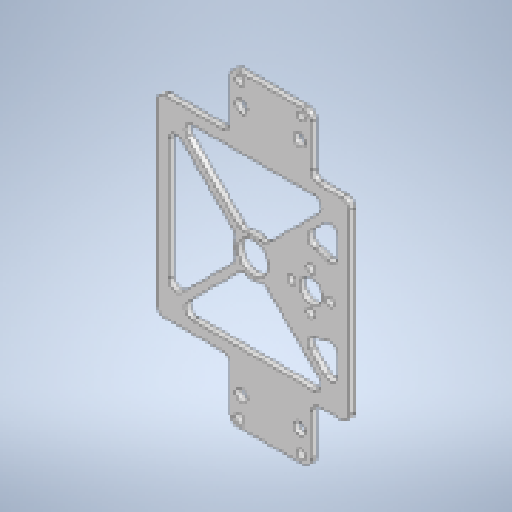
# Autodesk Inventor part: kataue
Saved by Autodesk Inventor 2025.1 (Build 291241000, 241)
## iProperties
Created: 2024-09-02
Part Number: kataue
Material: アルミニウム 2014-T4
Document SubType Name: Modeling
Designer: right
Density: 2.8 g/cm^3
Appearance: サテン
Mass: 6.17041 g
Surface Area: 41.087 cm^2
Volume: 2.20372 cm^3
Author: right
Autodesk Inventor part; units mm, degrees
ref_plane "YZ Plane" through (0, 0, 0) normal (1, 0, 0) x (0, 1, 0)
ref_plane "XZ Plane" through (0, 0, 0) normal (0, 1, 0) x (-1, 0, 0)
ref_plane "XY Plane" through (0, 0, 0) normal (0, 0, 1) x (1, 0, 0)
sketch "スケッチ1" plane through (0, 0, 0) normal (0, 0, 1) x (1, 0, 0)
  arc A0 (6.4508, -24.0185) -> (7.2151, -22.4459) centre (5.2151, -22.4459) ccw projected
  line L0 (7.2151, -22.4459) -> (7.2151, -18.7355) projected
  arc A1 (7.0743, -7.2531) -> (7.2151, -18.7355) centre (12.7151, -12.926) ccw projected
  arc A2 (7.0743, -7.2531) -> (2.2151, -6.426) centre (4.7151, -6.426) ccw projected
  line L1 (2.2151, -6.426) -> (2.2151, -154.426) projected
  arc A3 (2.2151, -154.426) -> (7.0743, -153.5989) centre (4.7151, -154.426) ccw projected
  arc A4 (7.2151, -142.1165) -> (7.0743, -153.5989) centre (12.7151, -147.926) ccw projected
  line L2 (7.2151, -142.1165) -> (7.2151, -138.4062) projected
  arc A5 (7.2151, -138.4062) -> (6.4508, -136.8336) centre (5.2151, -138.4062) ccw projected
  arc A6 (5.6865, -135.261) -> (6.4508, -136.8336) centre (7.6865, -135.261) ccw projected
  line L3 (5.6865, -135.261) -> (5.6865, -131.591) projected
  arc A7 (6.4508, -130.0185) -> (5.6865, -131.591) centre (7.6865, -131.591) ccw projected
  arc A8 (6.4508, -130.0185) -> (7.2151, -128.4459) centre (5.2151, -128.4459) ccw projected
  line L4 (7.2151, -128.4459) -> (7.2151, -122.426) projected
  arc A9 (9.2151, -120.426) -> (7.2151, -122.426) centre (9.2151, -122.426) ccw projected
  line L5 (9.2151, -120.426) -> (21.2151, -120.426) projected
  arc A10 (21.2151, -120.426) -> (23.2151, -118.426) centre (21.2151, -118.426) ccw projected
  line L6 (23.2151, -118.426) -> (23.2151, -42.426) projected
  arc A11 (23.2151, -42.426) -> (21.2151, -40.426) centre (21.2151, -42.426) ccw projected
  line L7 (21.2151, -40.426) -> (9.2151, -40.426) projected
  arc A12 (7.2151, -38.426) -> (9.2151, -40.426) centre (9.2151, -38.426) ccw projected
  line L8 (7.2151, -38.426) -> (7.2151, -32.4062) projected
  arc A13 (7.2151, -32.4062) -> (6.4508, -30.8336) centre (5.2151, -32.4062) ccw projected
  arc A14 (5.6865, -29.261) -> (6.4508, -30.8336) centre (7.6865, -29.261) ccw projected
  line L9 (5.6865, -29.261) -> (5.6865, -25.591) projected
  arc A15 (6.4508, -24.0185) -> (5.6865, -25.591) centre (7.6865, -25.591) ccw projected
  circle A16 centre (4.7151, -154.426) radius 1.1 projected
  circle A17 centre (4.7151, -6.426) radius 1.1 projected
  circle A18 centre (4.7151, -118.426) radius 1.1 projected
  circle A19 centre (20.7151, -42.426) radius 1.1 projected
  circle A20 centre (20.7151, -118.426) radius 1.1 projected
  circle A21 centre (4.7151, -42.426) radius 1.1 projected
  circle A22 centre (18.2151, -97.176) radius 1.1 projected
  circle A23 centre (7.2151, -63.676) radius 1.1 projected
  circle A24 centre (7.2151, -97.176) radius 1.1 projected
  circle A25 centre (18.2151, -63.676) radius 1.1 projected
  line L10 (9.2151, -40.426) -> (-0.7849, -40.426)
  line L11 (9.2151, -120.426) -> (-0.7849, -120.426)
  point P0 (0, 0)
  point P1 (4.7151, -154.426)
  point P2 (2.2151, -120.426)
  point P3 (2.2151, -40.426)
  constraints: 4 end point, 1 horizontal, 1 perpendicular, 1 tangent
extrude "押し出し1" add sketch "スケッチ1" along normal blind 1.5 contours L10 L7 A11 L6 A10 L5 L11 L1 | A22 | A23 | A24 | A25
sketch "スケッチ3" plane through (0, 0, 1.5) normal (0, 0, 1) x (1, 0, 0)
  line L0 (21.2151, -40.426) -> (2.2151, -40.426) projected
  line L1 (2.2151, -40.426) -> (2.2151, -120.426) projected
  line L2 (2.2151, -120.426) -> (21.2151, -120.426) projected
  arc A0 (21.2151, -120.426) -> (23.2151, -118.426) centre (21.2151, -118.426) ccw projected
  line L3 (23.2151, -118.426) -> (23.2151, -42.426) projected
  arc A1 (23.2151, -42.426) -> (21.2151, -40.426) centre (21.2151, -42.426) ccw projected
  circle A2 centre (4.7151, -42.426) radius 1.1 projected
  circle A3 centre (4.7151, -118.426) radius 1.1 projected
  circle A4 centre (20.7151, -118.426) radius 1.1 projected
  circle A5 centre (20.7151, -42.426) radius 1.1 projected
  line L4 (-16.7849, -57.426) -> (-16.7849, -103.426) projected
  line L5 (-14.7849, -105.426) -> (0.2151, -105.426) projected
  arc A6 (-16.7849, -103.426) -> (-14.7849, -105.426) centre (-14.7849, -103.426) ccw projected
  arc A7 (2.2151, -107.426) -> (0.2151, -105.426) centre (0.2151, -107.426) ccw projected
  arc A8 (0.2151, -55.426) -> (2.2151, -53.426) centre (0.2151, -53.426) ccw projected
  line L6 (0.2151, -55.426) -> (-14.7849, -55.426) projected
  arc A9 (-14.7849, -55.426) -> (-16.7849, -57.426) centre (-14.7849, -57.426) ccw projected
  arc A10 (25.2151, -105.426) -> (23.2151, -107.426) centre (25.2151, -107.426) ccw projected
  line L7 (25.2151, -105.426) -> (31.2151, -105.426) projected
  arc A11 (31.2151, -105.426) -> (33.2151, -103.426) centre (31.2151, -103.426) ccw projected
  line L8 (33.2151, -103.426) -> (33.2151, -57.426) projected
  line L9 (31.2151, -55.426) -> (25.2151, -55.426) projected
  arc A12 (33.2151, -57.426) -> (31.2151, -55.426) centre (31.2151, -57.426) ccw projected
  arc A13 (23.2151, -53.426) -> (25.2151, -55.426) centre (25.2151, -53.426) ccw projected
  point P0 (0, 0)
extrude "押し出し2" add sketch "スケッチ3" against normal up to surface (1.5 mm away) contours L1 A7 L5 A6 L4 A9 L6 A8 | A13 L9 A12 L8 A11 L7 A10 L3
fillet "フィレット2" radius 2 2 edges at (2.2151, -40.426, 0.75) (2.2151, -120.426, 0.75)
sketch "スケッチ4" plane through (0, 0, 1.5) normal (0, 0, 1) x (1, 0, 0)
  circle A0 centre (23.2151, -80.426) radius 10 construction
  line L0 (33.2151, -103.426) -> (33.2151, -57.426) projected
  circle A1 centre (23.2151, -80.426) radius 5 construction
  circle A2 centre (18.2151, -80.426) radius 1.1
  circle A3 centre (23.2151, -85.426) radius 1.1
  circle A4 centre (28.2151, -80.426) radius 1.1
  circle A5 centre (23.2151, -75.426) radius 1.1
  point P0 (0, 0)
  point P1 (33.2151, -80.426)
  dimension "d8" = 10
  dimension "d7" = 20
  dimension "d9" = 2.2
  dimension "d12" = 360
  constraints: 5 centre point, 3 horizontal alignment, 1 coincident, 1 midpoint, 1 tangent, 11 other
  measures "d7" diameter of A0
  measures "d9" diameter of A2
extrude "押し出し3" cut sketch "スケッチ4" against normal through all
sketch "スケッチ5" plane through (0, 0, 1.5) normal (0, 0, 1) x (1, 0, 0)
  circle A0 centre (5.2151, -47.926) radius 1.6 projected
  circle A1 centre (20.2151, -47.926) radius 1.6 projected
  circle A2 centre (5.2151, -112.926) radius 1.6 projected
  circle A3 centre (20.2151, -112.926) radius 1.6 projected
  point P0 (0, 0)
extrude "押し出し4" cut sketch "スケッチ5" against normal through all
sketch "スケッチ6" plane through (0, 0, 1.5) normal (0, 0, 1) x (1, 0, 0)
  circle A0 centre (23.2151, -80.426) radius 3 projected
  point P0 (0, 0)
extrude "押し出し5" cut sketch "スケッチ6" against normal through all
sketch "スケッチ7" plane through (0, 0, 1.5) normal (0, 0, 1) x (1, 0, 0)
  circle A0 centre (23.2151, -80.426) radius 3 projected
  circle A1 centre (5.2151, -47.926) radius 1.6 projected
  circle A2 centre (20.2151, -112.926) radius 1.6 projected
  circle A3 centre (20.2151, -47.926) radius 1.6 projected
  circle A4 centre (5.2151, -112.926) radius 1.6 projected
  circle A5 centre (28.2151, -80.426) radius 1.1 projected
  circle A6 centre (23.2151, -85.426) radius 1.1 projected
  circle A7 centre (18.2151, -80.426) radius 1.1 projected
  circle A8 centre (23.2151, -75.426) radius 1.1 projected
  arc A9 (2.2151, -118.426) -> (4.2151, -120.426) centre (4.2151, -118.426) ccw projected
  line L0 (4.2151, -120.426) -> (21.2151, -120.426) projected
  arc A10 (21.2151, -120.426) -> (23.2151, -118.426) centre (21.2151, -118.426) ccw projected
  line L1 (23.2151, -118.426) -> (23.2151, -107.426) projected
  arc A11 (25.2151, -105.426) -> (23.2151, -107.426) centre (25.2151, -107.426) ccw projected
  line L2 (25.2151, -105.426) -> (31.2151, -105.426) projected
  arc A12 (31.2151, -105.426) -> (33.2151, -103.426) centre (31.2151, -103.426) ccw projected
  line L3 (33.2151, -103.426) -> (33.2151, -57.426) projected
  arc A13 (33.2151, -57.426) -> (31.2151, -55.426) centre (31.2151, -57.426) ccw projected
  line L4 (31.2151, -55.426) -> (25.2151, -55.426) projected
  arc A14 (23.2151, -53.426) -> (25.2151, -55.426) centre (25.2151, -53.426) ccw projected
  line L5 (23.2151, -53.426) -> (23.2151, -42.426) projected
  arc A15 (23.2151, -42.426) -> (21.2151, -40.426) centre (21.2151, -42.426) ccw projected
  line L6 (21.2151, -40.426) -> (4.2151, -40.426) projected
  arc A16 (4.2151, -40.426) -> (2.2151, -42.426) centre (4.2151, -42.426) ccw projected
  line L7 (2.2151, -42.426) -> (2.2151, -53.426) projected
  arc A17 (0.2151, -55.426) -> (2.2151, -53.426) centre (0.2151, -53.426) ccw projected
  line L8 (0.2151, -55.426) -> (-14.7849, -55.426) projected
  arc A18 (-14.7849, -55.426) -> (-16.7849, -57.426) centre (-14.7849, -57.426) ccw projected
  line L9 (-16.7849, -57.426) -> (-16.7849, -103.426) projected
  arc A19 (-16.7849, -103.426) -> (-14.7849, -105.426) centre (-14.7849, -103.426) ccw projected
  line L10 (-14.7849, -105.426) -> (0.2151, -105.426) projected
  arc A20 (2.2151, -107.426) -> (0.2151, -105.426) centre (0.2151, -107.426) ccw projected
  line L11 (2.2151, -107.426) -> (2.2151, -118.426) projected
  circle A21 centre (4.7151, -42.426) radius 1.1 projected
  circle A22 centre (4.7151, -118.426) radius 1.1 projected
  circle A23 centre (20.7151, -118.426) radius 1.1 projected
  circle A24 centre (20.7151, -42.426) radius 1.1 projected
  circle A25 centre (23.2151, -80.426) radius 10
  line L12 (5.2151, -53.426) -> (5.2151, -43.426)
  line L13 (5.2151, -43.426) -> (20.2151, -43.426)
  line L14 (20.2151, -43.426) -> (20.2151, -53.426)
  arc A26 (20.2151, -53.426) -> (25.2151, -58.426) centre (25.2151, -53.426) ccw
  line L15 (25.2151, -58.426) -> (30.2151, -58.426)
  line L16 (30.2151, -58.426) -> (30.2151, -102.426)
  line L17 (30.2151, -102.426) -> (25.2151, -102.426)
  arc A27 (25.2151, -102.426) -> (20.2151, -107.426) centre (25.2151, -107.426) ccw
  line L18 (20.2151, -107.426) -> (20.2151, -117.426)
  line L19 (20.2151, -117.426) -> (5.2151, -117.426)
  line L20 (5.2151, -117.426) -> (5.2151, -107.426)
  arc A28 (5.2151, -107.426) -> (0.2151, -102.426) centre (0.2151, -107.426) ccw
  line L21 (0.2151, -102.426) -> (-13.7849, -102.426)
  line L22 (-13.7849, -102.426) -> (-13.7849, -58.426)
  line L23 (-13.7849, -58.426) -> (0.2151, -58.426)
  arc A29 (0.2151, -58.426) -> (5.2151, -53.426) centre (0.2151, -53.426) ccw
  line L24 (0.2151, -58.426) -> (25.2151, -58.426)
  line L25 (25.2151, -102.426) -> (0.2151, -102.426)
  line L26 (30.2151, -58.426) -> (-13.7849, -102.426) construction
  line L27 (30.2151, -102.426) -> (-13.7849, -58.426) construction
  circle A30 centre (8.2151, -80.426) radius 5
  circle A31 centre (8.2151, -80.426) radius 4
  line L28 (23.2151, -80.426) -> (8.2151, -80.426) construction
  line L29 (-12.3707, -58.426) -> (30.2151, -101.0118)
  line L30 (-13.7849, -59.8402) -> (28.8009, -102.426)
  line L31 (-12.3707, -102.426) -> (30.2151, -59.8402)
  line L32 (-13.7849, -101.0118) -> (28.8009, -58.426)
  point P0 (0, 0)
  point P1 (10.9721, -84.5972)
  point P2 (5.4581, -84.5972)
  point P3 (18.386, -89.1827)
  point P4 (30.2151, -87.5674)
  point P5 (18.386, -71.6693)
  point P6 (30.2151, -73.2846)
  point P7 (5.4581, -76.2548)
  point P8 (10.9721, -76.2548)
  point P9 (28.8009, -58.426)
  point P10 (4.0439, -83.183)
  point P11 (4.0439, -77.669)
  dimension "d20" = 3
  dimension "d21" = 8
  dimension "d22" = 1
  constraints: 42 end point, 8 point on circle, 7 centre point, 6 symmetric about line, 4 tangent, 3 parallel, 2 coincident, 2 point on line, 1 horizontal, 1 midpoint, 15 other
  measures "d20" radial gap between concentric circles of A17 A29
  measures "d21" diameter of A31
  measures "d22" distance between parallel lines of L27 L29
extrude "押し出し6" cut sketch "スケッチ7" against normal through all contours L24 L15 L32 A30 L29 L23 | L30 A30 L32 L22 | L29 L32 L30 A31 | A31 L32 L29 | A31 L31 L29 L32 | L30 L32 A31 | L29 L31 L30 L32 | L16 A25 L31 | A31 L29 L31 | A30 L30 L17 L25 L21 L31 | L32 L30 L31 A31 | L29 A31 L30 L31 | L31 L30 A31 | L16 L29 A25
fillet "フィレット3" radius 2 18 edges at (30.2151, -87.5674, 0.75) (30.2151, -101.0118, 0.75) (28.8009, -102.426, 0.75) (18.386, -89.1827, 0.75) (18.386, -71.6693, 0.75) (30.2151, -59.8402, 0.75) (30.2151, -73.2846, 0.75) (28.8009, -58.426, 0.75) (-12.3707, -102.426, 0.75) (-13.7849, -101.0118, 0.75) (5.4581, -84.5972, 0.75) (10.9721, -84.5972, 0.75) (10.9721, -76.2548, 0.75) (5.4581, -76.2548, 0.75) (4.0439, -77.669, 0.75) (4.0439, -83.183, 0.75) (-13.7849, -59.8402, 0.75) (-12.3707, -58.426, 0.75)
sketch "スケッチ8" plane through (0, 0, 1.5) normal (0, 0, 1) x (1, 0, 0)
  line L0 (8.2151, -105.426) -> (17.2151, -105.426)
  line L1 (17.2151, -105.426) -> (17.2151, -117.426)
  line L2 (17.2151, -117.426) -> (8.2151, -117.426)
  line L3 (8.2151, -117.426) -> (8.2151, -105.426)
  circle A0 centre (20.2151, -112.926) radius 1.6 projected
  circle A1 centre (5.2151, -112.926) radius 1.6 projected
  line L4 (4.2151, -120.426) -> (21.2151, -120.426) projected
  line L5 (23.9725, -102.426) -> (-7.5423, -102.426) projected
  line L6 (-16.7849, -57.426) -> (-16.7849, -103.426) construction
  line L7 (-16.7849, -80.426) -> (33.2151, -80.426) construction
  line L8 (33.2151, -103.426) -> (33.2151, -57.426) construction
  line L9 (8.2151, -55.426) -> (17.2151, -55.426)
  line L10 (17.2151, -55.426) -> (17.2151, -43.426)
  line L11 (17.2151, -43.426) -> (8.2151, -43.426)
  line L12 (8.2151, -43.426) -> (8.2151, -55.426)
  point P0 (0, 0)
  point P1 (5.2151, -47.926)
  dimension "d26" = 3
  dimension "d27" = 3
  dimension "d28" = 3
  dimension "d29" = 3
  constraints: 18 end point, 5 symmetric about line, 2 midpoint, 2 parallel, 1 horizontal, 1 perpendicular
  measures "d26" distance from line of A0.centre L1
  measures "d27" distance from line of A1.centre L3
  measures "d28" distance between parallel lines of L4 L2
  measures "d29" distance between parallel lines of L5 L0
extrude "押し出し7" cut sketch "スケッチ8" against normal through all contours L0 L1 L2 L3 | L12 L11 L10 L9
fillet "フィレット4" radius 2 8 edges at (17.2151, -105.426, 0.75) (8.2151, -105.426, 0.75) (8.2151, -117.426, 0.75) (17.2151, -117.426, 0.75) (8.2151, -55.426, 0.75) (17.2151, -55.426, 0.75) (17.2151, -43.426, 0.75) (8.2151, -43.426, 0.75)
equation "\"d26\" = d27"
equation "\"d28\" = d29"
